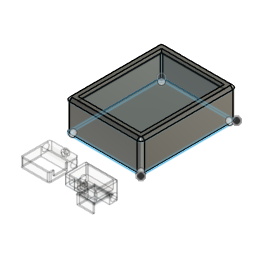
Hack PSU (Autodesk Fusion 360 design; units mm, degrees)
Autodesk Fusion 360 part; units mm, degrees
sketch "Sketch1" plane through (0, 0, 0) normal (0, 0, 1) x (1, 0, 0)
  line L0 (-17.5107, 11.2847) -> (3.4893, 11.2847)
  line L1 (3.4893, 11.2847) -> (3.4893, -3.2153)
  line L2 (3.4893, -3.2153) -> (-17.5107, -3.2153)
  line L3 (-17.5107, -3.2153) -> (-17.5107, 11.2847)
  line L4 (4.4893, -4.2153) -> (-18.5107, -4.2153)
  line L5 (-18.5107, -4.2153) -> (-18.5107, 12.2847)
  line L6 (-18.5107, 12.2847) -> (4.4893, 12.2847)
  line L7 (4.4893, 12.2847) -> (4.4893, -4.2153)
  line L8 (-18.5107, 12.2847) -> (4.4893, 12.2847)
  line L9 (4.4893, 12.2847) -> (4.4893, 19.2847)
  line L10 (4.4893, 19.2847) -> (-18.5107, 19.2847)
  line L11 (-18.5107, 19.2847) -> (-18.5107, 12.2847)
  dimension "d1" = 14.5
  dimension "d2" = 21
  dimension "d3" = -1
  dimension "d4" = 7
  constraint horizontal L0
  constraint vertical L1
  constraint horizontal L2
  constraint vertical L3
  constraint horizontal L8
  constraint vertical L9
  constraint horizontal L10
  constraint vertical L11
  measures "d1" distance of L0.start L2.end
  measures "d2" distance of L0.start L0.end
  measures "d4" distance of L5.end L10.end
extrude "Extrude1" add sketch "Sketch1" along normal blind 7 makes body 1
sketch "Sketch2" plane through (4.4893, 0, 0) normal (1, 0, 0) x (0, 1, 0)
  line L0 (-4.2153, 0) -> (19.2847, 0)
  line L1 (19.2847, 0) -> (19.2847, 7)
  line L2 (19.2847, 7) -> (-4.2153, 7)
  line L3 (-4.2153, 7) -> (-4.2153, 0)
  circle A0 centre (15.7847, 3.5) radius 2.75
  line L4 (15.7847, 3.5) -> (15.7847, 7) construction
  line L5 (15.7847, 3.5) -> (19.2847, 3.5) construction
  line L6 (15.7847, 3.5) -> (15.7847, 0) construction
  line L7 (-0.2153, 7) -> (9.7847, 7)
  line L8 (9.7847, 7) -> (9.7847, 3)
  line L9 (9.7847, 3) -> (-0.2153, 3)
  line L10 (-0.2153, 3) -> (-0.2153, 7)
  dimension "d7" = 5.5
  dimension "d22" = 10
  dimension "d23" = 4
  dimension "d24" = 4
  constraint coincident A0.centre L4.start
  constraint coincident L2 L4.end
  constraint perpendicular L2 L4
  constraint midpoint L1 L5.end
  constraint coincident L0 L6.end
  constraint perpendicular L0 L6
  constraint equal L4 L5
  constraint equal L5 L6
  constraint horizontal L7
  constraint vertical L8
  constraint horizontal L9
  constraint vertical L10
  constraint coincident L2 L7.start
  measures "d7" diameter of A0
  measures "d22" distance of L8.end L9.end
  measures "d23" distance of L7.start L9.end
  measures "d24" distance of L3 L10
extrude "Extrude2" cut sketch "Sketch2" against normal blind 30 contours A0 bodies 1
sketch "Sketch3" plane through (0, 19.2847, 0) normal (0, 1, 0) x (-1, 0, 0)
  line L0 (-4.4893, 0) -> (18.5107, 0)
  line L1 (18.5107, 0) -> (18.5107, 7)
  line L2 (18.5107, 7) -> (-4.4893, 7)
  line L3 (-4.4893, 7) -> (-4.4893, 0)
  circle A0 centre (7.0107, 3.4168) radius 1.5
  line L4 (7.0107, 3.4168) -> (7.0107, 7) construction
  line L5 (7.0107, 3.4168) -> (7.0107, 0) construction
  circle A1 centre (7.0107, 3.4168) radius 2.5
  dimension "d10" = 3
  dimension "d13" = 5
  constraint coincident A0.centre L4.start
  constraint midpoint L2 L4.end
  constraint midpoint L0 L5.end
  constraint perpendicular L0 L5
  constraint parallel L4 L5
  constraint concentric A0 A1
  measures "d10" diameter of A0
  measures "d13" diameter of A1
extrude "Extrude3" cut sketch "Sketch3" against normal blind 3 contours A0 bodies 1
extrude "Extrude4" add sketch "Sketch3" along normal blind 2 contours A1 bodies 1
fillet "Fillet1" radius 1.5 2 edges at (-18.5107, -4.2153, 3.5) (4.4893, -4.2153, 3.5) on bodies 1
fillet "Fillet2" radius 1.5 1 edges at (4.4893, 19.2847, 3.5) on bodies 1
fillet "Fillet3" radius 1.5 1 edges at (-18.5107, 19.2847, 3.5) on bodies 1
extrude "Extrude5" cut sketch "Sketch2" against normal blind 5 contours L2 L7 L8 L9 L10 bodies 1
sketch "Sketch4" plane through (0, 0, 0) normal (0, 0, 1) x (1, 0, 0)
  line L0 (20.2781, 10.1951) -> (41.2781, 10.1951)
  line L1 (41.2781, 10.1951) -> (41.2781, -3.8049)
  line L2 (41.2781, -3.8049) -> (20.2781, -3.8049)
  line L3 (20.2781, -3.8049) -> (20.2781, 10.1951)
  line L4 (43.2781, -5.8049) -> (18.2781, -5.8049)
  line L5 (18.2781, -5.8049) -> (18.2781, 12.1951)
  line L6 (18.2781, 12.1951) -> (43.2781, 12.1951)
  line L7 (43.2781, 12.1951) -> (43.2781, -5.8049)
  line L8 (18.2781, 12.1951) -> (43.2781, 12.1951)
  line L9 (43.2781, 12.1951) -> (43.2781, 5.1951)
  line L10 (43.2781, 5.1951) -> (18.2781, 5.1951)
  line L11 (18.2781, 5.1951) -> (18.2781, 12.1951)
  dimension "d27" = 21
  dimension "d28" = 14
  dimension "d29" = -2
  dimension "d30" = 7
  constraint horizontal L0
  constraint vertical L1
  constraint horizontal L2
  constraint vertical L3
  constraint horizontal L8
  constraint vertical L9
  constraint horizontal L10
  constraint vertical L11
  constraint coincident L7 L9.end
  measures "d27" distance of L0.start L0.end
  measures "d28" distance of L0.start L2.end
  measures "d30" distance of L6 L10
extrude "Extrude6" add sketch "Sketch4" along normal blind 14 separate body contours L0 L1 L3 L5 L6 L7 L8 L9 L10 L11 | L0 L1 L3 L10 | L1 L2 L3 L4 L5 L7 L10 makes body 2
extrude "Extrude7" cut sketch "Sketch4" along normal blind 7 contours L1 L2 L3 L4 L5 L7 L10 bodies 2
extrude "Extrude8" cut sketch "Sketch4" along normal blind 7 and the other way blind -14 contours L0 L1 L3 L10 bodies 2
sketch "Sketch5" plane through (43.2781, 0, 0) normal (1, 0, 0) x (0, 1, 0)
  line L0 (-5.8049, 7) -> (5.1951, 7)
  line L1 (5.1951, 7) -> (5.1951, 0)
  line L2 (5.1951, 0) -> (12.1951, 0)
  line L3 (12.1951, 0) -> (12.1951, 14)
  line L4 (12.1951, 14) -> (-5.8049, 14)
  line L5 (-5.8049, 14) -> (-5.8049, 7)
  circle A0 centre (8.6951, 3.5) radius 2.75
  line L6 (8.6951, 3.5) -> (8.6951, 0) construction
  line L7 (8.6951, 3.5) -> (5.1951, 3.5) construction
  line L8 (8.6951, 3.5) -> (12.1951, 3.5) construction
  dimension "d39" = 5.5
  constraint coincident A0.centre L6.start
  constraint midpoint L2 L6.end
  constraint coincident L1 L7.end
  constraint perpendicular L1 L7
  constraint equal L6 L7
  constraint coincident L3 L8.end
  constraint perpendicular L3 L8
  constraint equal L6 L8
  measures "d39" diameter of A0
extrude "Extrude9" cut sketch "Sketch5" against normal blind 28 contours A0 bodies 2
sketch "Sketch6" plane through (0, 5.1951, 0) normal (0, -1, 0) x (1, 0, 0)
  line L0 (41.2781, 7) -> (20.2781, 7)
  line L1 (20.2781, 7) -> (18.2781, 7)
  line L2 (18.2781, 7) -> (18.2781, 0)
  line L3 (18.2781, 0) -> (43.2781, 0)
  line L4 (43.2781, 0) -> (43.2781, 7)
  line L5 (43.2781, 7) -> (41.2781, 7)
  circle A0 centre (23.2781, 3.5004) radius 1.5
  circle A1 centre (23.2781, 3.5004) radius 2.5
  line L6 (18.2781, 0) -> (28.2781, 0)
  line L7 (28.2781, 0) -> (28.2781, 7)
  line L8 (28.2781, 7) -> (18.2781, 7)
  line L9 (18.2781, 7) -> (18.2781, 0)
  dimension "d42" = 3
  dimension "d45" = 5
  dimension "d48" = 20
  dimension "d56" = 10
  constraint concentric A0 A1
  constraint horizontal L6
  constraint vertical L7
  constraint horizontal L8
  constraint vertical L9
  constraint coincident L2.end L3.start
  measures "d42" diameter of A0
  measures "d45" diameter of A1
  measures "d48" distance of L4 A0.centre
  measures "d56" distance of L2.end L6.end
extrude "Extrude10" cut sketch "Sketch6" against normal blind 2 contours A0 bodies 2
extrude "Extrude11" add sketch "Sketch6" along normal blind 2 contours A1 bodies 2
sketch "Sketch8" plane through (0, 0, 7) normal (0, 0, -1) x (1, 0, 0)
  line L0 (43.2781, -5.1951) -> (43.2781, 5.8049)
  line L1 (43.2781, 5.8049) -> (18.2781, 5.8049)
  line L2 (18.2781, 5.8049) -> (18.2781, -5.1951)
  line L3 (18.2781, -5.1951) -> (20.2781, -5.1951)
  line L4 (20.2781, -5.1951) -> (20.2781, 3.8049)
  line L5 (20.2781, 3.8049) -> (41.2781, 3.8049)
  line L6 (41.2781, 3.8049) -> (41.2781, -5.1951)
  line L7 (41.2781, -5.1951) -> (43.2781, -5.1951)
  line L8 (43.2781, -5.1951) -> (31.2781, -5.1951)
  line L9 (31.2781, -5.1951) -> (31.2781, 6.8049)
  line L10 (31.2781, 6.8049) -> (43.2781, 6.8049)
  line L11 (43.2781, 6.8049) -> (43.2781, -5.1951)
  line L12 (44.2781, -6.1951) -> (30.2781, -6.1951)
  line L13 (30.2781, -6.1951) -> (30.2781, 7.8049)
  line L14 (30.2781, 7.8049) -> (44.2781, 7.8049)
  line L15 (44.2781, 7.8049) -> (44.2781, -6.1951)
  line L16 (43.2781, 6.8049) -> (43.2781, 7.8049)
  line L17 (43.2781, -5.1951) -> (43.2781, -6.1951)
  line L18 (31.2781, -5.1951) -> (30.2781, -5.1951)
  dimension "d49" = 12
  dimension "d50" = 12
  dimension "d51" = -1
  constraint horizontal L8
  constraint vertical L9
  constraint horizontal L10
  constraint vertical L11
  constraint coincident L0.start L7.end
  constraint coincident L14 L16.end
  constraint perpendicular L14 L16
  constraint coincident L12 L17.end
  constraint perpendicular L12 L17
  constraint coincident L13 L18.end
  constraint perpendicular L13 L18
  measures "d49" distance of L0.start L10.end
  measures "d50" distance of L9.end L10.end
extrude "Extrude12" add sketch "Sketch8" against normal blind 1 contours L1 L9 L10 L11 | L1 L9 L10 L13 L14 L16 bodies 2
extrude "Extrude13" add sketch "Sketch8" along normal blind 7 contours L1 L5 L9 L13 | L1 L9 L10 L13 L14 L16 | L5 L9 L13 L18 bodies 2
move_face "OffsetFaces1" offset 2 1 faces at (28.7781, 5.1951, 3.5001) on bodies 2
move_face "OffsetFaces2" offset 2 1 faces at (28.4448, 3.1951, 3.5001) on bodies 2
sketch "Sketch9" plane through (0, 0, 0) normal (0, 0, -1) x (1, 0, 0)
  line L0 (30.2781, -1.1951) -> (18.2781, -1.1951)
  line L1 (18.2781, -1.1951) -> (18.2781, -12.1951)
  line L2 (18.2781, -12.1951) -> (43.2781, -12.1951)
  line L3 (43.2781, -12.1951) -> (43.2781, -5.1951)
  line L4 (43.2781, -5.1951) -> (31.2781, -5.1951)
  line L5 (31.2781, -5.1951) -> (31.2781, 6.8049)
  line L6 (31.2781, 6.8049) -> (43.2781, 6.8049)
  line L7 (43.2781, 6.8049) -> (43.2781, 7.8049)
  line L8 (43.2781, 7.8049) -> (30.2781, 7.8049)
  line L9 (30.2781, 7.8049) -> (30.2781, -1.1951)
  line L10 (20.5281, -2.4708) -> (26.0281, -2.4708)
  line L11 (26.0281, -2.4708) -> (26.0281, -4.9708)
  line L12 (26.0281, -4.9708) -> (20.5281, -4.9708)
  line L13 (20.5281, -4.9708) -> (20.5281, -2.4708)
  dimension "d59" = 5.5
  dimension "d60" = 2.5
  dimension "d61" = 2.25
  constraint horizontal L10
  constraint vertical L11
  constraint horizontal L12
  constraint vertical L13
  measures "d59" distance of L11.end L12.end
  measures "d60" distance of L10.start L12.end
  measures "d61" distance of L1 L13
extrude "Extrude14" cut sketch "Sketch9" against normal blind 7 contours L10 L11 L12 L13 bodies 2
chamfer "Chamfer1" distance 1 angle 45 9 edges at (43.2781, 12.1951, 7) (18.2781, -5.8049, 10.5) (18.2781, 12.1951, 7) (18.2781, 1.1951, 3.5) (30.7781, 12.1951, 0) (30.7781, 12.1951, 14) (30.7781, -5.8049, 14) (43.2781, -5.8049, 11) (43.2781, 3.1951, 14) on bodies 2
sketch "Sketch1 (2)" plane through (0, 0, 0) normal (0, 0, 1) x (1, 0, 0) in component "Component"
  line L0 (-21.0301, 114.0253) -> (32.9699, 114.0253)
  line L1 (35.9699, 111.0253) -> (35.9699, 40.5253)
  line L2 (32.9699, 37.5253) -> (-21.0301, 37.5253)
  line L3 (-24.0301, 40.5253) -> (-24.0301, 111.0253)
  arc A0 (-21.0301, 114.0253) -> (-24.0301, 111.0253) centre (-21.0301, 111.0253) ccw
  arc A1 (35.9699, 111.0253) -> (32.9699, 114.0253) centre (32.9699, 111.0253) ccw
  arc A2 (32.9699, 37.5253) -> (35.9699, 40.5253) centre (32.9699, 40.5253) ccw
  arc A3 (-24.0301, 40.5253) -> (-21.0301, 37.5253) centre (-21.0301, 40.5253) ccw
  line L4 (33.9699, 111.0253) -> (33.9699, 40.5253)
  arc A4 (32.9699, 39.5253) -> (33.9699, 40.5253) centre (32.9699, 40.5253) ccw
  line L5 (32.9699, 39.5253) -> (-21.0301, 39.5253)
  arc A5 (-22.0301, 40.5253) -> (-21.0301, 39.5253) centre (-21.0301, 40.5253) ccw
  line L6 (-22.0301, 40.5253) -> (-22.0301, 111.0253)
  arc A6 (-21.0301, 112.0253) -> (-22.0301, 111.0253) centre (-21.0301, 111.0253) ccw
  line L7 (-21.0301, 112.0253) -> (32.9699, 112.0253)
  arc A7 (33.9699, 111.0253) -> (32.9699, 112.0253) centre (32.9699, 111.0253) ccw
  point P0 (-24.0301, 114.0253)
  point P1 (35.9699, 114.0253)
  point P2 (35.9699, 37.5253)
  dimension "d65" = 60
  dimension "d66" = 76.5
  dimension "d67" = 2
  dimension "d72" = 3
  constraint horizontal L0
  constraint vertical L1
  constraint horizontal L2
  constraint vertical L3
  constraint coincident P0 L0
  constraint coincident P0 L3
  constraint tangent L0 A0
  constraint tangent L3 A0
  constraint coincident P1 L0
  constraint coincident P1 L1
  constraint tangent L0 A1
  constraint tangent L1 A1
  constraint equal A0 A1
  constraint coincident P2 L1
  constraint coincident P2 L2
  constraint tangent L1 A2
  constraint tangent L2 A2
  constraint equal A0 A2
  constraint tangent L2 A3
  constraint tangent L3 A3
  constraint equal A0 A3
  measures "d65" distance of P0 P1
  measures "d66" distance of P1 P2
  measures "d72" radius of A0
extrude "Extrude1'" add sketch "Sketch1 (2)" along normal blind 2 separate body contours L0 L1 L2 L3 A0 A1 A2 A3 | L4 A4 L5 A5 L6 A6 L7 A7 makes body 3 in component "Component"
extrude "Extrude2'" add sketch "Sketch1 (2)" along normal blind 22 bodies 3 in component "Component"
chamfer "Chamfer1'" distance 1 angle 45 1 faces at (15.9699, 64.0253, 0) on bodies 3 in component "Component"
sketch "Sketch2 (2)" plane through (0, 0, 22) normal (0, 0, 1) x (-1, 0, 0) in component "Component"
  arc A0 (-32.9699, -39.5253) -> (-33.9699, -40.5253) centre (-32.9699, -40.5253) ccw
  line L0 (-32.9699, -39.5253) -> (21.0301, -39.5253)
  arc A1 (22.0301, -40.5253) -> (21.0301, -39.5253) centre (21.0301, -40.5253) ccw
  line L1 (22.0301, -40.5253) -> (22.0301, -111.0253)
  arc A2 (21.0301, -112.0253) -> (22.0301, -111.0253) centre (21.0301, -111.0253) ccw
  line L2 (21.0301, -112.0253) -> (-32.9699, -112.0253)
  arc A3 (-33.9699, -111.0253) -> (-32.9699, -112.0253) centre (-32.9699, -111.0253) ccw
  line L3 (-33.9699, -111.0253) -> (-33.9699, -40.5253)
  arc A4 (21.0301, -114.0253) -> (24.0301, -111.0253) centre (21.0301, -111.0253) ccw
  line L4 (24.0301, -111.0253) -> (24.0301, -40.5253)
  arc A5 (24.0301, -40.5253) -> (21.0301, -37.5253) centre (21.0301, -40.5253) ccw
  line L5 (21.0301, -37.5253) -> (-32.9699, -37.5253)
  arc A6 (-32.9699, -37.5253) -> (-35.9699, -40.5253) centre (-32.9699, -40.5253) ccw
  line L6 (-35.9699, -40.5253) -> (-35.9699, -111.0253)
  arc A7 (-35.9699, -111.0253) -> (-32.9699, -114.0253) centre (-32.9699, -111.0253) ccw
  line L7 (-32.9699, -114.0253) -> (21.0301, -114.0253)
  line L8 (19.0301, -109.0253) -> (-30.9699, -109.0253)
  line L9 (19.0301, -42.5253) -> (19.0301, -109.0253)
  line L10 (-30.9699, -42.5253) -> (19.0301, -42.5253)
  line L11 (-30.9699, -109.0253) -> (-30.9699, -42.5253)
  dimension "d74" = 3
extrude "Extrude3'" add sketch "Sketch2 (2)" along normal blind 3 contours A0 L0 A1 L1 A2 L2 A3 L3 | A4 L4 A5 L5 A6 L6 A7 L7 bodies 3 in component "Component"
chamfer "Chamfer2" distance 2 angle 45 8 edges at (5.9699, 37.5253, 25) (35.0912, 38.4039, 25) (35.9699, 75.7753, 25) (35.0912, 113.1466, 25) (5.9699, 114.0253, 25) (-23.1514, 113.1466, 25) (-24.0301, 75.7753, 25) (-23.1514, 38.4039, 25) on bodies 3 in component "Component"
chamfer "Chamfer3" distance 1 angle 45 8 edges at (5.9699, 39.5253, 22) (-21.7372, 39.8181, 22) (-22.0301, 75.7753, 22) (-21.7372, 111.7324, 22) (5.9699, 112.0253, 22) (33.677, 111.7324, 22) (33.9699, 75.7753, 22) (33.677, 39.8181, 22) on bodies 3 in component "Component"
component "Component" placed x (1, 0, 0) y (0, 1, 0) z (0, 0, 1) at (0, 0, 0)
